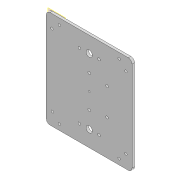
# Autodesk Inventor part: fechamentocima
Saved by Autodesk Inventor 2020 (Build 240168000, 168)
## iProperties
Created: 2022-07-23
Part Number: fechamentocima
Material: Genérico
Document SubType Name: Modeling
Designer: gabri
Density: 1 g/cm^3
Appearance: Padrão
Author: gabri
Autodesk Inventor part; units mm, degrees
ref_plane "YZ Plane" through (0, 0, 0) normal (1, 0, 0) x (0, 1, 0)
ref_plane "XZ Plane" through (0, 0, 0) normal (0, 1, 0) x (-1, 0, 0)
ref_plane "XY Plane" through (0, 0, 0) normal (0, 0, 1) x (1, 0, 0)
ref_plane "Plano de trabalho1" through (0, 142, 0) normal (0, 0, 1) x (0, -1, 0)
sketch "Esboço1" plane through (0, 142, 0) normal (0, 0, 1) x (0, -1, 0)
  arc A0 (124, -4) -> (125, -5) centre (125, -4) ccw projected
  line L0 (142, -5) -> (125, -5) projected
  line L1 (142, -5) -> (142, -8) projected
  line L2 (142, -8) -> (144, -8) projected
  arc A1 (144, -8) -> (150, -2) centre (144, -2) ccw projected
  line L3 (150, -2) -> (150, 0) projected
  line L4 (150, 0) -> (147, 0) projected
  line L5 (147, 0) -> (147, 17) projected
  arc A2 (147, 17) -> (146, 18) centre (146, 17) ccw projected
  line L6 (135, 18) -> (146, 18) projected
  arc A3 (135, 18) -> (134, 17) centre (135, 17) ccw projected
  line L7 (134, 9) -> (134, 17) projected
  arc A4 (133, 8) -> (134, 9) centre (133, 9) ccw projected
  line L8 (133, 8) -> (124, 8) projected
  line L9 (124, -4) -> (124, 8) projected
  circle A5 centre (141, 13) radius 2 projected
  circle A6 centre (129, 2) radius 2 projected
  arc A7 (-4, 18) -> (-5, 17) centre (-4, 17) ccw projected
  line L10 (-5, 0) -> (-5, 17) projected
  line L11 (-5, 0) -> (-8, 0) projected
  line L12 (-8, 0) -> (-8, -2) projected
  arc A8 (-8, -2) -> (-2, -8) centre (-2, -2) ccw projected
  line L13 (-2, -8) -> (0, -8) projected
  line L14 (0, -8) -> (0, -5) projected
  line L15 (0, -5) -> (17, -5) projected
  arc A9 (17, -5) -> (18, -4) centre (17, -4) ccw projected
  line L16 (18, 7) -> (18, -4) projected
  arc A10 (18, 7) -> (17, 8) centre (17, 7) ccw projected
  line L17 (9, 8) -> (17, 8) projected
  arc A11 (8, 9) -> (9, 8) centre (9, 9) ccw projected
  line L18 (8, 9) -> (8, 18) projected
  line L19 (-4, 18) -> (8, 18) projected
  circle A12 centre (13, 1) radius 2 projected
  circle A13 centre (2, 13) radius 2 projected
  circle A14 centre (141, 110) radius 2 projected
  circle A15 centre (129, 121) radius 2 projected
  arc A16 (146, 105) -> (147, 106) centre (146, 106) ccw projected
  line L20 (147, 123) -> (147, 106) projected
  line L21 (150, 123) -> (147, 123) projected
  line L22 (150, 125) -> (150, 123) projected
  arc A17 (150, 125) -> (144, 131) centre (144, 125) ccw projected
  line L23 (144, 131) -> (124, 131) projected
  line L24 (124, 116) -> (124, 131) projected
  arc A18 (124, 116) -> (125, 115) centre (125, 116) ccw projected
  line L25 (133, 115) -> (125, 115) projected
  arc A19 (134, 114) -> (133, 115) centre (133, 114) ccw projected
  line L26 (134, 114) -> (134, 106) projected
  arc A20 (134, 106) -> (135, 105) centre (135, 106) ccw projected
  line L27 (146, 105) -> (135, 105) projected
  arc A21 (17, 115) -> (18, 116) centre (17, 116) ccw projected
  line L28 (18, 131) -> (18, 116) projected
  line L29 (-2, 131) -> (18, 131) projected
  arc A22 (-2, 131) -> (-8, 125) centre (-2, 125) ccw projected
  line L30 (-8, 125) -> (-8, 123) projected
  line L31 (-8, 123) -> (-5, 123) projected
  line L32 (-5, 123) -> (-5, 106) projected
  arc A23 (-5, 106) -> (-4, 105) centre (-4, 106) ccw projected
  line L33 (7, 105) -> (-4, 105) projected
  arc A24 (7, 105) -> (8, 106) centre (7, 106) ccw projected
  line L34 (8, 114) -> (8, 106) projected
  arc A25 (9, 115) -> (8, 114) centre (9, 114) ccw projected
  line L35 (9, 115) -> (17, 115) projected
  circle A26 centre (1, 110) radius 2 projected
  circle A27 centre (13, 121) radius 2 projected
  line L36 (18, 131) -> (124.2929, 131)
  line L37 (150, 123) -> (150, 0)
  line L38 (0, -8) -> (142, -8)
  line L39 (-8, 0) -> (-8, 123)
  point P0 (142, 0)
  constraints: 8 end point, 3 perpendicular, 1 point on line
extrude "Extrusão1" add sketch "Esboço1" along normal blind 4
sketch "Esboço2" plane through (0, 142, 4) normal (0, 0, 1) x (1, 0, 0)
  circle A0 centre (61.5, -17.9015) radius 5 projected
  circle A1 centre (61.5, -124.1015) radius 5 projected
  circle A2 centre (61.5038, -71.0015) radius 5.8 projected
  circle A3 centre (61.5, -45.0015) radius 2.1 projected
  circle A4 centre (61.5, -97.0015) radius 2.1 projected
  circle A5 centre (61.5, -17.9015) radius 5.05
  circle A6 centre (61.5, -45.0015) radius 2.1
  circle A7 centre (61.5, -97.0015) radius 2.1
  circle A8 centre (61.5038, -71.0015) radius 1.5
  circle A9 centre (61.5, -124.1015) radius 5
  point P0 (0, -142)
  dimension "d2" = 10.1
  dimension "d3" = 4.2
  dimension "d4" = 3
  dimension "d19" = 10
  constraints: 5 centre point, 5 coincident, 2 concentric
  measures "d2" diameter of A5
  measures "d3" diameter of A6
  measures "d4" diameter of A8
  measures "d19" diameter of A1
extrude "Extrusão2" cut sketch "Esboço2" against normal blind 4 contours A0 | A1 | A3 | A4 | A8
sketch "Esboço3" plane through (0, 142, 4) normal (0, 0, 1) x (1, 0, 0)
  circle A0 centre (61.5, -124.1015) radius 5 projected
  circle A1 centre (61.5, -124.1015) radius 16
  circle A2 centre (61.5, -17.9015) radius 5 projected
  circle A3 centre (61.5, -17.9015) radius 16
  line L0 (45.5, -17.9015) -> (77.5, -17.9015)
  line L1 (45.5, -124.1015) -> (77.5, -124.1015)
  circle A4 centre (77.5, -124.1015) radius 2.1
  circle A5 centre (45.5, -124.1015) radius 2.1
  circle A6 centre (77.5, -17.9015) radius 2.1
  circle A7 centre (45.5, -17.9015) radius 2.1
  point P0 (0, -142)
  dimension "d7" = 32
  dimension "d8" = 32
  dimension "d9" = 4.2
  dimension "d10" = 4.2
  dimension "d11" = 4.2
  dimension "d12" = 4.2
  constraints: 6 centre point, 6 coincident, 4 end point, 4 point on circle, 1 horizontal, 1 parallel
  measures "d7" diameter of A1
  measures "d8" diameter of A3
  measures "d9" diameter of A4
  measures "d10" diameter of A5
  measures "d11" diameter of A6
  measures "d12" diameter of A7
extrude "Extrusão3" cut sketch "Esboço3" against normal blind 4 contours A4 A1 L1 | L1 A1 A4 | A5 A1 L1 | L1 A1 A5 | A1 A4 | A1 A5 | A6 A3 L0 | L0 A3 A6 | A7 A3 L0 | L0 A3 A7 | A3 A6 | A3 A7
sketch "Esboço4" plane through (0, 142, 0) normal (0, 0, -1) x (-1, 0, 0)
  circle A0 centre (-90.5, -93.0015) radius 2.1
  circle A1 centre (-90.5, -49.0015) radius 2.1
  point P0 (0, -142)
  dimension "d15" = 4.2
  dimension "d16" = 4.2
  constraints: 2 centre point
  measures "d15" diameter of A0
  measures "d16" diameter of A1
extrude "Extrusão4" cut sketch "Esboço4" against normal blind 4
sketch "Esboço5" plane through (0, 142, 4) normal (0, 0, 1) x (1, 0, 0)
  circle A0 centre (61.5, -124.1015) radius 5 projected
  circle A1 centre (61.5, -124.1015) radius 5.05
  circle A2 centre (61.5, -17.9015) radius 5 projected
  circle A3 centre (61.5, -17.9015) radius 5.05
  point P0 (0, -142)
  dimension "d20" = 10.1
  dimension "d21" = 10.1
  constraints: 2 centre point, 2 coincident
  measures "d20" diameter of A1
  measures "d21" diameter of A3
extrude "Extrusão5" cut sketch "Esboço5" against normal blind 10
